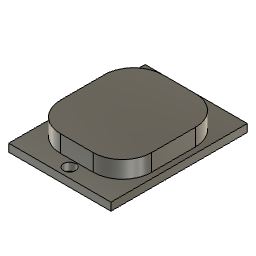
PMW3360 v1 (Autodesk Fusion 360 design; units mm, degrees)
Autodesk Fusion 360 part; units mm, degrees
sketch "Sketch1" plane through (0, 0, 0) normal (0, 0, 1) x (1, 0, 0)
  line L0 (0, 0) -> (0, 28) construction
  line L1 (0, 28) -> (21, 28) construction
  line L2 (21, 28) -> (0, 28) construction
  line L3 (0, 28) -> (0, 0) construction
  line L4 (0, 0) -> (21, 0) construction
  line L5 (21, 0) -> (21, 28) construction
  line L6 (10.5, 0) -> (10.5, 28) construction
  line L7 (10.5, 0) -> (10.5, 2) construction
  line L8 (10.5, 28) -> (10.5, 26) construction
  circle A0 centre (10.5, 26) radius 1.25 construction
  circle A1 centre (10.5, 2) radius 1.25 construction
  line L9 (21, 28) -> (0, 28)
  line L10 (0, 28) -> (0, 0)
  line L11 (0, 0) -> (21, 0)
  line L12 (21, 0) -> (21, 28)
  circle A2 centre (10.5, 2) radius 1.25
  circle A3 centre (10.5, 26) radius 1.25
  dimension "d38" = 28
  dimension "d39" = 21
  dimension "d40" = 2
  dimension "d41" = 2
  dimension "d42" = 2.5
  dimension "d43" = 2.5
  constraint coincident L0.start L3.end
  constraint vertical L0
  constraint perpendicular L0 L1
  constraint horizontal L2
  constraint vertical L3
  constraint horizontal L4
  constraint vertical L5
  constraint midpoint L4 L6.start
  constraint midpoint L2 L6.end
  constraint perpendicular L4 L7
  constraint perpendicular L1 L8
  constraint coincident L8.end A0.centre
  constraint coincident L7.end A1.centre
  constraint horizontal L9
  constraint vertical L10
  constraint horizontal L11
  constraint vertical L12
  constraint concentric A1 A2
  constraint concentric A0 A3
  measures "d38" distance of L0.start L0.end
  measures "d39" distance of L0.end L1.end
  measures "d40" distance of L6.start L7.end
  measures "d41" distance of L6.end L8.end
  measures "d42" diameter of A0
  measures "d43" diameter of A1
extrude "Extrude1" add sketch "Sketch1" along normal blind 1.6
sketch "Sketch2" plane through (0, 0, 1.6) normal (0, 0, 1) x (-1, 0, 0)
  circle A0 centre (-10.5, -26) radius 1.25
  circle A1 centre (-10.5, -2) radius 1.25
  line L0 (-21, 0) -> (-21, -28)
  line L1 (-21, -28) -> (0, -28)
  line L2 (0, -28) -> (0, 0)
  line L3 (0, 0) -> (-21, 0)
  line L4 (0, -14) -> (-21, -14) construction
  line L5 (-10.5, -28) -> (-10.5, 0) construction
  line L6 (-10.5, -14) -> (-10.5, -24.5) construction
  line L7 (-10.5, -24.5) -> (-19.85, -24.5) construction
  line L8 (-10.5, -14) -> (-10.5, -3.5) construction
  line L9 (-10.5, -3.5) -> (-1.15, -3.5) construction
  line L10 (-1.15, -3.5) -> (-19.85, -3.5) construction
  line L11 (-19.85, -3.5) -> (-19.85, -24.5) construction
  line L12 (-19.85, -24.5) -> (-1.15, -24.5) construction
  line L13 (-1.15, -24.5) -> (-1.15, -3.5) construction
  line L14 (-1.15, -3.5) -> (-19.85, -3.5)
  line L15 (-19.85, -3.5) -> (-19.85, -24.5)
  line L16 (-19.85, -24.5) -> (-1.15, -24.5)
  line L17 (-1.15, -24.5) -> (-1.15, -3.5)
  dimension "d46" = 10.5
  dimension "d47" = 9.35
  dimension "d48" = 10.5
  dimension "d49" = 9.35
  constraint midpoint L2 L4.start
  constraint midpoint L0 L4.end
  constraint midpoint L1 L5.start
  constraint midpoint L3 L5.end
  constraint midpoint L5 L6.start
  constraint perpendicular L4 L6
  constraint perpendicular L6 L7
  constraint perpendicular L7 L8
  constraint perpendicular L5 L9
  constraint horizontal L10
  constraint vertical L11
  constraint horizontal L12
  constraint vertical L13
  constraint horizontal L14
  constraint vertical L15
  constraint horizontal L16
  constraint vertical L17
  measures "d46" distance of L6.start L6.end
  measures "d47" distance of L6.end L7.end
  measures "d48" distance of L6.start L8.end
  measures "d49" distance of L8.end L9.end
extrude "Extrude2" add sketch "Sketch2" along normal blind 3.5 contours L14 L15 L16 L17
fillet "Fillet1" radius 6 4 edges at (19.85, 3.5, 3.35) (1.15, 3.5, 3.35) (1.15, 24.5, 3.35) (19.85, 24.5, 3.35)
